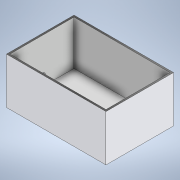
# Autodesk Inventor part: cajaEléctrica
Saved by Autodesk Inventor 2020 (Build 240168000, 168)
## iProperties
Created: 2021-10-16
Part Number: cajaEléctrica
Material: Genérico
Document SubType Name: Modeling
Designer: DANIEL
Density: 1 g/cm^3
Appearance: Valor por defecto
Author: DANIEL
Autodesk Inventor part; units mm, degrees
ref_plane "YZ Plane" through (0, 0, 0) normal (1, 0, 0) x (0, 1, 0)
ref_plane "XZ Plane" through (0, 0, 0) normal (0, 1, 0) x (-1, 0, 0)
ref_plane "XY Plane" through (0, 0, 0) normal (0, 0, 1) x (1, 0, 0)
sketch "Boceto1" plane through (0, 0, 0) normal (0, 1, 0) x (-1, 0, 0)
  line L0 (140, 95) -> (-140, 95)
  line L1 (-140, 95) -> (-140, -95)
  line L2 (-140, -95) -> (140, -95)
  line L3 (140, -95) -> (140, 95)
  point P0 (0, 0)
  dimension "d0" = 280
  dimension "d1" = 190
  dimension "d2" = 95
  dimension "d3" = 140
  constraints: 8 end point, 2 parallel, 1 horizontal, 1 perpendicular
  measures "d0" distance between parallel lines of L1 L3
  measures "d1" distance between parallel lines of L2 L0
  measures "d2" distance from line of L0 point (0, 0)
  measures "d3" distance from line of point (0, 0) L1
extrude "Extrusión1" add sketch "Boceto1" along normal blind 130
ref_plane "Plano de trabajo1" through (0, 0, 95) normal (1, 0, 0) x (0, 0, -1)
ref_plane "Plano de trabajo2" through (140, 0, 0) normal (0, 0, -1) x (-1, 0, 0)
sketch "Boceto3" plane through (0, 130, 0) normal (0, 1, 0) x (1, 0, 0)
  line L0 (140, 95) -> (-140, 95) projected
  line L1 (-140, 95) -> (-140, -95) projected
  line L2 (-140, -95) -> (140, -95) projected
  line L3 (140, -95) -> (140, 95) projected
  line L4 (-135, -90) -> (135, -90)
  line L5 (135, -90) -> (135, 90)
  line L6 (135, 90) -> (-135, 90)
  line L7 (-135, 90) -> (-135, -90)
  point P0 (0, 0)
  dimension "d7" = 270
  dimension "d8" = 135
  dimension "d9" = 180
  dimension "d10" = 90
  constraints: 8 end point, 2 parallel, 1 horizontal, 1 perpendicular
  measures "d7" distance between parallel lines of L5 L7
  measures "d8" distance from line of L7 point (0, 0)
  measures "d9" distance between parallel lines of L6 L4
  measures "d10" distance from line of L4 point (0, 0)
extrude "Extrusión2" cut sketch "Boceto3" against normal blind 125 contours L7 L6 L5 L4
sketch "Boceto4" plane through (-140, 0, -95) normal (-1, 0, 0) x (0, 0, 1)
  circle A0 centre (95, 29.1709) radius 10
  point P0 (95, 0)
  dimension "d13" = 20
  constraints: 1 centre point
  measures "d13" diameter of A0
extrude "Extrusión3" cut sketch "Boceto4" against normal blind 5
sketch "Boceto6" plane through (0, 130, 0) normal (0, 1, 0) x (1, 0, 0)
  line L0 (-140, -95) -> (140, -95) projected
  line L1 (-140, 95) -> (-140, -95) projected
  line L2 (140, 95) -> (-140, 95) projected
  line L3 (140, -95) -> (140, 95) projected
  line L4 (-140, -95) -> (140, -95)
  line L5 (140, -95) -> (140, 95)
  line L6 (140, 95) -> (-140, 95)
  line L7 (-140, 95) -> (-140, -95)
  point P0 (0, 0)
  constraints: 8 end point, 2 parallel, 1 horizontal, 1 perpendicular
extrude "Extrusión4" [suppressed]
